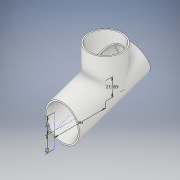
# Autodesk Inventor part: auger
Saved by Autodesk Inventor 2019 (Build 230136000, 136)
## iProperties
Created: 2019-01-23
Part Number: auger
Material: Generic
Document SubType Name: Modeling
Designer: jmc
Density: 1 g/cm^3
Appearance: PET White_1
Author: jmc
Autodesk Inventor part; units mm, degrees
ref_plane "YZ Plane" through (0, 0, 0) normal (1, 0, 0) x (0, 1, 0)
ref_plane "XZ Plane" through (0, 0, 0) normal (0, 1, 0) x (-1, 0, 0)
sketch "Sketch2" plane through (0, 0, 0) normal (0, 1, 0) x (-1, 0, 0)
  circle A0 centre (0, 0) radius 27
  dimension "d1" = 54
  constraints: 1 centre point, 1 coincident
  measures "d1" diameter of A0
extrude "Extrusion1" add sketch "Sketch2" along normal blind 80
sketch "Sketch3" plane through (0, 0, 0) normal (1, 0, 0) x (0, 1, 0)
  line L0 (0, 0) -> (0, 80) construction
  line L1 (0, 27) -> (0, -27) construction
  line L2 (0, 80) -> (25, 80) construction
  line L3 (0, 80) -> (-25, 80) construction
  line L4 (0, 80) -> (39.583, -33.2594) construction
  line L5 (0, 0) -> (27.9592, 0) construction
  line L6 (51.5233, -67.4244) -> (27.9592, 0) construction
  line L7 (27.9592, 0) -> (-12.5, 115.7665) construction
  dimension "d4" = 80
  dimension "d5" = 25
  dimension "d6" = 25
  dimension "d14" = 27.9592
  constraints: 14 end point, 3 horizontal, 1 collinear, 1 point on line
  measures "d4" distance of L0.start L0.end
  measures "d5" distance of L0.end L2.end
  measures "d6" distance of L0.end L3.end
  measures "d14" distance of L5.end L0.start
ref_plane "Work Plane1" through (0, 0, 80) normal (0, 0.3299211, -0.9440085) x (-1, 0, 0)
sketch "Sketch5" plane through (0, 0, 80) normal (0, 0.3299211, -0.9440085) x (-1, 0, 0)
  circle A0 centre (0, 0) radius 27
  point P0 (0, -26.3937)
  dimension "d9" = 54
  constraints: 1 centre point
  measures "d9" diameter of A0
extrude "Extrusion2" add sketch "Sketch5" along normal blind 130 and the other way blind 10 separate body
ref_plane "Work Plane2" through (0, 27.9592, 0) normal (0, -1, 0) x (1, 0, 0)
sketch "Sketch7" plane through (0, 27.9592, 0) normal (0, -1, 0) x (1, 0, 0)
  circle A0 centre (0, 0) radius 27 projected
extrude "corte de la parte baja del tubo vertical" cut sketch "Sketch7" along normal up to next bodies 1
shell "Shell1" thickness 2 removed faces 2 at (-5.1126, 7.7594, 93.305) at (7.506, 80, 12.3045) bodies 2 1
sketch "Sketch8" plane through (0, 0, 80) normal (0, 0.3299211, -0.9440085) x (-1, 0, 0)
  circle A0 centre (0, 0) radius 25 projected
  point P0 (0, -26.3937)
extrude "corte horizontal (vaciado del tubo)" cut sketch "Sketch8" along normal blind 125 bodies 2 1
sketch "Sketch9" plane through (0, 80, 0) normal (0, 1, 0) x (1, 0, 0)
  circle A0 centre (0, 0) radius 25 projected
extrude "corte vertical (vaciado del tubo)" cut sketch "Sketch9" against normal up to surface (52.0408 mm away) bodies 2
sketch "Sketch10" plane through (0, 42.8897, -42.7211) normal (0, 0.3299211, -0.9440085) x (-1, 0, 0)
  circle A0 centre (0, 0) radius 3
  point P0 (0, -26.3937)
  dimension "d23" = 6
  constraints: 1 centre point, 1 coincident
  measures "d23" diameter of A0
extrude "Extrusion6" cut sketch "Sketch10" against normal up to next bodies 2
ref_plane "Work Plane3" through (0, 7.4328, 58.7324) normal (0, -0.3299211, 0.9440085) x (1, 0, 0)
sketch "medida del tubo horizontal" plane through (0, 0, 0) normal (1, 0, 0) x (0, 1, 0)
  line L0 (22.189, 98.348) -> (-28.7874, 80.5322) projected
  line L1 (17.4015, -51.629) -> (68.378, -33.8132) projected
  line L2 (63.8782, -27) -> (63.1792, -25) projected
  line L3 (63.1792, -25) -> (80, -25) projected
  line L4 (80, -25) -> (80, -27) projected
  line L5 (80, -27) -> (63.8782, -27) projected
  line L6 (45.7047, 25) -> (45.0058, 27) projected
  line L7 (45.0058, 27) -> (80, 27) projected
  line L8 (80, 27) -> (80, 25) projected
  line L9 (80, 25) -> (45.7047, 25) projected
  line L10 (63.1792, -25) -> (65.2978, -25) projected
  line L11 (65.2978, -25) -> (68.378, -33.8132) projected
  line L12 (68.378, -33.8132) -> (45.7218, -41.7313) projected
  line L13 (45.7218, -41.7313) -> (45.0619, -39.8433) projected
  line L14 (45.0619, -39.8433) -> (65.8301, -32.5851) projected
  line L15 (65.8301, -32.5851) -> (63.1792, -25) projected
  line L16 (47.8234, 25) -> (45.7047, 25) projected
  line L17 (45.7047, 25) -> (20.301, 97.6881) projected
  line L18 (20.301, 97.6881) -> (22.189, 98.348) projected
  line L19 (22.189, 98.348) -> (47.8234, 25) projected
  line L20 (-26.8994, 81.1921) -> (18.6297, -49.0811) projected
  line L21 (18.6297, -49.0811) -> (39.3979, -41.8229) projected
  line L22 (39.3979, -41.8229) -> (40.0577, -43.7109) projected
  line L23 (40.0577, -43.7109) -> (17.4015, -51.629) projected
  line L24 (17.4015, -51.629) -> (-28.7874, 80.5322) projected
  line L25 (-28.7874, 80.5322) -> (-26.8994, 81.1921) projected
  line L26 (63.8782, -27) -> (63.1792, -25) projected
  line L27 (63.1792, -25) -> (80, -25) projected
  line L28 (80, -25) -> (80, -27) projected
  line L29 (80, -27) -> (63.8782, -27) projected
  line L30 (45.7047, 25) -> (45.0058, 27) projected
  line L31 (45.0058, 27) -> (80, 27) projected
  line L32 (80, 27) -> (80, 25) projected
  line L33 (80, 25) -> (45.7047, 25) projected
  line L34 (63.1792, -25) -> (65.2978, -25) projected
  line L35 (65.2978, -25) -> (68.378, -33.8132) projected
  line L36 (68.378, -33.8132) -> (45.7218, -41.7313) projected
  line L37 (45.7218, -41.7313) -> (45.0619, -39.8433) projected
  line L38 (45.0619, -39.8433) -> (65.8301, -32.5851) projected
  line L39 (65.8301, -32.5851) -> (63.1792, -25) projected
  line L40 (47.8234, 25) -> (45.7047, 25) projected
  line L41 (45.7047, 25) -> (20.301, 97.6881) projected
  line L42 (20.301, 97.6881) -> (22.189, 98.348) projected
  line L43 (22.189, 98.348) -> (47.8234, 25) projected
  line L44 (-26.8994, 81.1921) -> (18.6297, -49.0811) projected
  line L45 (18.6297, -49.0811) -> (39.3979, -41.8229) projected
  line L46 (39.3979, -41.8229) -> (40.0577, -43.7109) projected
  line L47 (40.0577, -43.7109) -> (17.4015, -51.629) projected
  line L48 (17.4015, -51.629) -> (-28.7874, 80.5322) projected
  line L49 (-28.7874, 80.5322) -> (-26.8994, 81.1921) projected
  line L50 (63.8782, -27) -> (63.1792, -25) projected
  line L51 (63.1792, -25) -> (80, -25) projected
  line L52 (80, -25) -> (80, -27) projected
  line L53 (80, -27) -> (63.8782, -27) projected
  line L54 (45.7047, 25) -> (45.0058, 27) projected
  line L55 (45.0058, 27) -> (80, 27) projected
  line L56 (80, 27) -> (80, 25) projected
  line L57 (80, 25) -> (45.7047, 25) projected
  line L58 (63.1792, -25) -> (65.2978, -25) projected
  line L59 (65.2978, -25) -> (68.378, -33.8132) projected
  line L60 (68.378, -33.8132) -> (45.7218, -41.7313) projected
  line L61 (45.7218, -41.7313) -> (45.0619, -39.8433) projected
  line L62 (45.0619, -39.8433) -> (65.8301, -32.5851) projected
  line L63 (65.8301, -32.5851) -> (63.1792, -25) projected
  line L64 (47.8234, 25) -> (45.7047, 25) projected
  line L65 (45.7047, 25) -> (20.301, 97.6881) projected
  line L66 (20.301, 97.6881) -> (22.189, 98.348) projected
  line L67 (22.189, 98.348) -> (47.8234, 25) projected
  line L68 (-26.8994, 81.1921) -> (18.6297, -49.0811) projected
  line L69 (18.6297, -49.0811) -> (39.3979, -41.8229) projected
  line L70 (39.3979, -41.8229) -> (40.0577, -43.7109) projected
  line L71 (40.0577, -43.7109) -> (17.4015, -51.629) projected
  line L72 (17.4015, -51.629) -> (-28.7874, 80.5322) projected
  line L73 (-28.7874, 80.5322) -> (-26.8994, 81.1921) projected
  line L74 (-94.9364, 22.9555) -> (120.6645, 98.3057) projected
  line L75 (63.8782, -27) -> (63.1792, -25) projected
  line L76 (63.1792, -25) -> (80, -25) projected
  line L77 (80, -25) -> (80, -27) projected
  line L78 (80, -27) -> (63.8782, -27) projected
  line L79 (45.7047, 25) -> (45.0058, 27) projected
  line L80 (45.0058, 27) -> (80, 27) projected
  line L81 (80, 27) -> (80, 25) projected
  line L82 (80, 25) -> (45.7047, 25) projected
  line L83 (63.1792, -25) -> (65.2978, -25) projected
  line L84 (65.2978, -25) -> (68.378, -33.8132) projected
  line L85 (68.378, -33.8132) -> (45.7218, -41.7313) projected
  line L86 (45.7218, -41.7313) -> (45.0619, -39.8433) projected
  line L87 (45.0619, -39.8433) -> (65.8301, -32.5851) projected
  line L88 (65.8301, -32.5851) -> (63.1792, -25) projected
  line L89 (47.8234, 25) -> (45.7047, 25) projected
  line L90 (45.7047, 25) -> (20.301, 97.6881) projected
  line L91 (20.301, 97.6881) -> (22.189, 98.348) projected
  line L92 (22.189, 98.348) -> (47.8234, 25) projected
  line L93 (-26.8994, 81.1921) -> (18.6297, -49.0811) projected
  line L94 (18.6297, -49.0811) -> (39.3979, -41.8229) projected
  line L95 (39.3979, -41.8229) -> (40.0577, -43.7109) projected
  line L96 (40.0577, -43.7109) -> (17.4015, -51.629) projected
  line L97 (17.4015, -51.629) -> (-28.7874, 80.5322) projected
  line L98 (-28.7874, 80.5322) -> (-26.8994, 81.1921) projected
  line L99 (22.189, 98.348) -> (68.378, -33.8132) projected
  line L100 (32.921, 67.6403) -> (-24.2819, 67.6403)
  point P0 (0, 0)
  dimension "d26" = 140
  constraints: 3 point on line, 2 end point, 1 coincident, 1 horizontal
  measures "d26" distance between parallel lines of L1 L0
ref_plane "Work Plane4" through (0, -24.2819, 67.6403) normal (0, 0, 1) x (1, 0, 0)
split "Split1" plane through (0, -24.2819, 67.6403) removes the side toward (0, 0, 1) bodies 2
body "Solid4"
body "Solid2"
